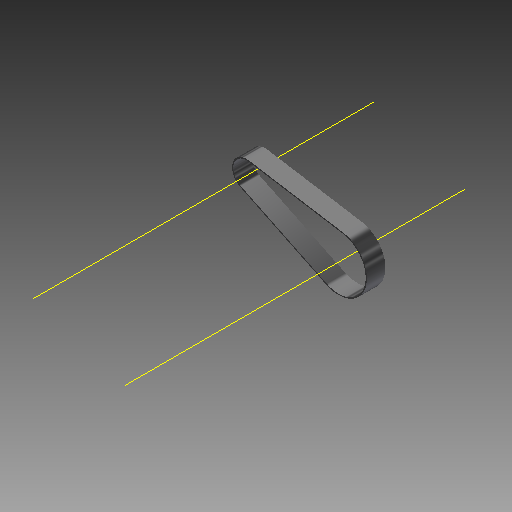
# Autodesk Inventor part: Synchronous Belt
Saved by Autodesk Inventor 2019.4 (Build 234330000, 330)
## iProperties
Created: 2020-01-16
Part Number: Synchronous Belt
Material: Rubber
Document SubType Name: Modeling
Designer: admin
Density: 0.93 g/cm^3
Appearance: Rubber - Black - Version 1.1
Mass: 3.7944 g
Surface Area: 86.7 cm^2
Volume: 4.08 cm^3
CustomPartVersion: 1
Author: admin
Autodesk Inventor part; units mm, degrees
sketch "Sketch Path" plane through (0, 0, 0) normal (0, 0, 1) x (1, 0, 0)
  arc A0 (-152.1931, -35.9008) -> (-159.3081, -58.4283) centre (-154.1115, -47.6823) ccw
  arc A1 (-85.4644, -94.1384) -> (-71.2343, -49.0834) centre (-75.0711, -72.6463) ccw
  line L0 (-85.4644, -94.1384) -> (-159.3081, -58.4283)
  line L1 (-152.1931, -35.9008) -> (-71.2343, -49.0834)
  constraints: 4 end point, 4 point on circle, 2 centre point
ref_plane "Cross Section Plane" through (-159.3081, -58.4283, 0) normal (0.9003, -0.4354, 0) x (0, 0, 1)
ref_plane "Work Plane2" through (-154.1115, -47.6823, 0) normal (-1, 0, 0) x (0, 0, 1)
ref_plane "Work Plane3" through (-75.0711, -72.6463, 0) normal (-0.979, 0.2039, 0) x (0, 0, 1)
sketch "Cross Section" plane through (-159.3081, -58.4283, 0) normal (0.9003, -0.4354, 0) x (0, 0, 1)
  line L0 (-8, 0.5) -> (8, 0.5)
  line L1 (8, 0.5) -> (8, -0.5)
  line L2 (8, -0.5) -> (-8, -0.5)
  line L3 (-8, -0.5) -> (-8, 0.5)
  line L4 (-8, 0) -> (8, 0) construction
  point P0 (0, 0)
  point P1 (0, 0)
  dimension "d0" = 16
  dimension "d4" = 0.5
  dimension "d5" = 0.5
  constraints: 10 end point, 3 midpoint, 2 parallel, 1 coincident, 1 horizontal, 1 perpendicular, 1 other
  measures "d0" distance between parallel lines of L1 L3
  measures "d4" distance between parallel lines of L2 L4
  measures "d5" distance between parallel lines of L4 L0
sweep "Belt" add profiles "Cross Section" path "Sketch Path"
equation "\"d0\" = da_B"
equation "\"d4\" = da_a"
equation "\"d5\" = da_a2"
equation "\"da_B\" = 16"
equation "\"da_pb\" = 5"
equation "\"da_L\" = 279.99995"
equation "\"da_a\" = 0.5"
equation "\"da_S\" = 2.65"
equation "\"da_Beta\" = 20deg"
equation "\"da_Ht\" = 1.2"
equation "\"da_H\" = 2.2"
equation "\"da_a2\" = 0.5"
body "Solid1"
